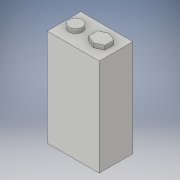
# Autodesk Inventor part: Pile
Saved by Autodesk Inventor 2019 (Build 230136000, 136)
## iProperties
Created: 2020-05-13
Part Number: Pile
Material: Générique
Document SubType Name: Modeling
Designer: Quentin
Density: 1 g/cm^3
Appearance: Par défaut
Author: Quentin
Autodesk Inventor part; units mm, degrees
ref_plane "YZ Plane" through (0, 0, 0) normal (1, 0, 0) x (0, 1, 0)
ref_plane "XZ Plane" through (0, 0, 0) normal (0, 1, 0) x (-1, 0, 0)
ref_plane "XY Plane" through (0, 0, 0) normal (0, 0, 1) x (1, 0, 0)
sketch "Esquisse1" plane through (0, 0, 0) normal (0, 0, 1) x (1, 0, 0)
  line L0 (0, 0) -> (0, 47.5)
  line L1 (0, 47.5) -> (25.5, 47.5)
  line L2 (25.5, 47.5) -> (25.5, 0)
  line L3 (25.5, 0) -> (0, 0)
  dimension "d0" = 47.5
  dimension "d1" = 25.5
  constraints: 8 end point, 3 perpendicular, 1 vertical
  measures "d0" distance of L0.start L0.end
  measures "d1" distance of L0.end L1.end
extrude "Extrusion1" add sketch "Esquisse1" along normal blind 16.5
sketch "Esquisse2" plane through (0, 47.5, 0) normal (0, 1, 0) x (1, 0, 0)
  line L0 (0, 0) -> (0, -16.5) projected
  line L1 (25.5, 0) -> (25.5, -16.5) projected
  circle A0 centre (5.753, -8.25) radius 3.25
  line L2 (25.5, -8.25) -> (18.2294, -8.25)
  line L3 (14.2294, -8.25) -> (14.2294, -6.05)
  line L4 (14.2294, -8.25) -> (14.2294, -10.45)
  line L5 (22.2294, -8.25) -> (22.2294, -6.05)
  line L6 (22.2294, -8.25) -> (22.2294, -10.45)
  line L7 (22.2294, -10.45) -> (18.2294, -12.25)
  line L8 (18.2294, -12.25) -> (14.2294, -10.45)
  line L9 (14.2294, -6.05) -> (18.2294, -4.25)
  line L10 (18.2294, -4.25) -> (22.2294, -6.05)
  dimension "d4" = 6.5
  dimension "d6" = 2.2
  dimension "d7" = 2.2
  dimension "d8" = 2.2
  dimension "d9" = 2.2
  constraints: 18 end point, 3 vertical, 1 centre point, 1 horizontal, 1 midpoint, 1 perpendicular, 1 point on line
  measures "d4" diameter of A0
  measures "d6" distance of L3.start L3.end
  measures "d7" distance of L3.start L4.end
  measures "d8" distance of L5.start L5.end
  measures "d9" distance of L5.start L6.end
extrude "Extrusion2" add sketch "Esquisse2" along normal blind 2
